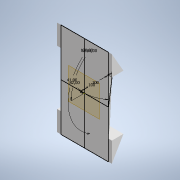
# Autodesk Inventor part: camera_vision
Saved by Autodesk Inventor 2022 (Build 260153000, 153)
## iProperties
Created: 2024-11-25
Part Number: camera_vision
Material: Типовые
Document SubType Name: Modeling
Designer: Andrey
Density: 1 g/cm^3
Appearance: По умолчанию
Author: Andrey
Autodesk Inventor part; units mm, degrees
ref_plane "YZ Plane" through (0, 0, 0) normal (1, 0, 0) x (0, 1, 0)
ref_plane "XZ Plane" through (0, 0, 0) normal (0, 1, 0) x (-1, 0, 0)
sketch "Эскиз1" plane through (0, 0, 0) normal (0, 1, 0) x (-1, 0, 0)
  line L0 (0, 0) -> (0, 100)
  line L1 (0, 0) -> (-173.2051, 100)
  line L2 (-173.2051, 100) -> (173.2051, 100)
  line L3 (173.2051, 100) -> (0, 0)
  dimension "d0" = 120
  dimension "d1" = 60
  dimension "d5" = 100
  constraints: 8 end point, 1 midpoint, 1 perpendicular, 1 vertical
  measures "d0" angle of L3 L1
  measures "d1" angle of L3 L0
  measures "d5" distance of L0.start L0.end
sketch "Эскиз2" plane through (0, 0, 0) normal (1, 0, 0) x (0, 1, 0)
  line L0 (0, 0) -> (0, 100)
  line L1 (-173.2051, 100) -> (173.2051, 100)
  line L2 (173.2051, 100) -> (0, 0)
  line L3 (0, 0) -> (-173.2051, 100)
  dimension "d2" = 120
  dimension "d3" = 60
  dimension "d6" = 100
  constraints: 8 end point, 1 horizontal, 1 midpoint, 1 perpendicular, 1 vertical
  measures "d2" angle of L2 L3
  measures "d3" angle of L2 L0
  measures "d6" distance of L0.start L0.end
ref_plane "РабПлоскость1" through (0, 0, 100) normal (0, 0, 1) x (1, 0, 0)
sketch "Эскиз3" plane through (0, 0, 100) normal (0, 0, 1) x (1, 0, 0)
  line L0 (-173.2051, -173.2051) -> (173.2051, -173.2051)
  line L1 (173.2051, -173.2051) -> (173.2051, 173.2051)
  line L2 (173.2051, 173.2051) -> (-173.2051, 173.2051)
  line L3 (-173.2051, 173.2051) -> (-173.2051, -173.2051)
  line L4 (173.2051, 0) -> (-173.2051, 0) projected
  line L5 (0, -173.2051) -> (0, 173.2051) projected
  point P0 (0, 0)
  constraints: 8 end point, 4 midpoint, 2 parallel, 1 horizontal, 1 perpendicular
sketch "Эскиз4" plane through (0, 0, 0) normal (1, 0, 0) x (0, 1, 0)
  line L0 (173.2051, 100) -> (0, 0) projected
  line L1 (0, 0) -> (-173.2051, 100) projected
  line L2 (173.2051, 100) -> (-173.2051, 100) projected
extrude "Выдавливание1" add sketch "Эскиз4" along normal mid plane 500
sketch "Эскиз5" plane through (0, 0, 0) normal (0, 1, 0) x (-1, 0, 0)
  line L0 (250, 0) -> (-250, 0) projected
  line L1 (-250, 100) -> (-250, 0) projected
  line L2 (-250, 100) -> (250, 100) projected
  line L3 (250, 0) -> (250, 100) projected
  line L4 (173.2051, 100) -> (0, 0) projected
  line L5 (0, 0) -> (-173.2051, 100) projected
  point P0 (-100, 57.735)
  point P1 (100, 57.735)
extrude "Выдавливание2" cut sketch "Эскиз5" along normal mid plane 800 contours L0 L4 L2 L3 | L0 L1 L2 L5
equation "\"d1\" = 0.5 * d0"
equation "\"d3\" = 0.5 * d2"
